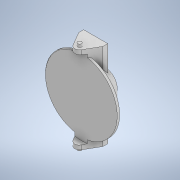
# Autodesk Inventor part: B_axis
Saved by Autodesk Inventor 2020 (Build 240168000, 168)
## iProperties
Created: 2020-05-02
Part Number: B_axis
Material: Generic
Document SubType Name: Modeling
Designer: zhang
Density: 1 g/cm^3
Appearance: Default
Author: zhang
Autodesk Inventor part; units mm, degrees
ref_plane "YZ Plane" through (0, 0, 0) normal (1, 0, 0) x (0, 1, 0)
ref_plane "XZ Plane" through (0, 0, 0) normal (0, 1, 0) x (-1, 0, 0)
ref_plane "XY Plane" through (0, 0, 0) normal (0, 0, 1) x (1, 0, 0)
sketch "Sketch1" plane through (0, 0, 0) normal (0, 1, 0) x (-1, 0, 0)
  line L0 (289.4755, 0) -> (-215.021, 0)
  line L1 (0, 324.0308) -> (0, -320.0636)
  circle A0 centre (0, 0) radius 10 construction
  line L2 (17.3205, 10) -> (50, -46.6025)
  line L3 (50, -46.6025) -> (0, -46.6025) construction
  line L4 (-17.3205, 10) -> (-50, -46.6025)
  line L5 (-50, -46.6025) -> (0, -46.6025) construction
  arc A1 (17.3205, 10) -> (-17.3205, 10) centre (0, 0) ccw
  line L6 (50, -46.6025) -> (50, -66.6025)
  line L7 (50, -66.6025) -> (-50, -66.6025)
  line L8 (-50, -66.6025) -> (-50, -46.6025)
  point P0 (0, 40)
  dimension "d0" = 20
  dimension "d1" = 50
  dimension "d2" = 60
  dimension "d3" = 40
  dimension "d4" = 20
  dimension "d5" = 20
  constraints: 18 end point, 4 point on line, 3 perpendicular, 3 vertical, 2 centre point, 2 horizontal, 2 point on circle, 2 tangent, 1 coincident, 1 symmetric about line
  measures "d0" diameter of A0
  measures "d1" distance of L2.end L3.end
  measures "d2" angle of L3 L2
  measures "d3" distance of point (0, 0) point (0, 40)
  measures "d4" radius of A1
  measures "d5" distance of L2.end L6.end
extrude "Extrusion1" add sketch "Sketch1" along normal mid plane 360
sketch "Sketch2" plane through (0, 0, 0) normal (0, 1, 0) x (-1, 0, 0)
  line L0 (0, 66.6254) -> (0, -94.0572)
  line L1 (109.0661, 0) -> (-97.6998, 0)
  line L2 (0, -6) -> (150, -6)
  line L3 (150, -6) -> (150, -16)
  line L4 (150, -16) -> (140, -16)
  line L5 (140, -16) -> (50, -106)
  line L6 (50, -106) -> (0, -106)
  line L7 (0, -106) -> (0, -6)
  point P0 (0, 0)
  point P1 (0, -94.0572)
  dimension "d8" = 150
  dimension "d9" = 12
  dimension "d10" = 135
  dimension "d11" = 50
  dimension "d12" = 100
  dimension "d13" = 10
  constraints: 16 end point, 3 horizontal, 2 perpendicular, 2 vertical, 1 collinear, 1 parallel, 1 point on line
  measures "d8" distance of L2.start L2.end
  measures "d9" diameter of L2 L1
  measures "d10" angle of L6 L5
  measures "d11" distance of L5.end L6.end
  measures "d12" distance of L6.end L2.start
  measures "d13" distance of L2.end L3.end
revolve "Revolution1" add sketch "Sketch2" angle 360 about axis through (0, 0, 66.6254) along (0, 0, -1)
sketch "Sketch3" plane through (0, 0, -6) normal (0, 0, 1) x (1, 0, 0)
  circle A0 centre (0, 0) radius 163
  dimension "d15" = 326
  constraints: 1 centre point, 1 coincident
  measures "d15" diameter of A0
extrude "Extrusion2" cut sketch "Sketch3" along normal blind 360
sketch "Sketch4" plane through (0, 180, 0) normal (0, 1, 0) x (1, 0, 0)
  circle A0 centre (0, 0) radius 8
  dimension "d18" = 16
  constraints: 1 centre point, 1 coincident
  measures "d18" diameter of A0
extrude "Extrusion3" add sketch "Sketch4" along normal blind 12
mirror "Mirror1" about plane through (0, 0, 0) normal (0, 1, 0) of "Extrusion3"
chamfer "Chamfer1" distance 2 angle 45 2 edges at (-150, 0, -6) (-150, 0, -16)
body "Solid1"
